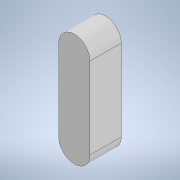
# Autodesk Inventor part: Motor_key
Saved by Autodesk Inventor 2020 (Build 240168000, 168)
## iProperties
Created: 2022-06-09
Part Number: Motor_key
Material: 일반
Document SubType Name: Modeling
Designer: samsung
Density: 1 g/cm^3
Appearance: 기본값
Author: samsung
Autodesk Inventor part; units mm, degrees
ref_plane "YZ Plane" through (0, 0, 0) normal (1, 0, 0) x (0, 1, 0)
ref_plane "XZ Plane" through (0, 0, 0) normal (0, 1, 0) x (-1, 0, 0)
ref_plane "XY Plane" through (0, 0, 0) normal (0, 0, 1) x (1, 0, 0)
sketch "스케치1" plane through (0, 0, 0) normal (0, 0, 1) x (1, 0, 0)
  line L0 (5, 0) -> (5, -15.5) projected
  line L1 (0, 0) -> (5, 0) projected
  line L2 (0, 0) -> (0, -15.5) projected
  arc A0 (0, -15.5) -> (5, -15.5) centre (2.5, -15.5) ccw projected
  arc A1 (5, -2.5) -> (0, -2.5) centre (2.5, -2.5) ccw
  constraints: 2 point on circle, 2 point on line, 1 centre point, 1 tangent
extrude "돌출1" add sketch "스케치1" along normal blind 5 contours L0 A0 L2 A1
